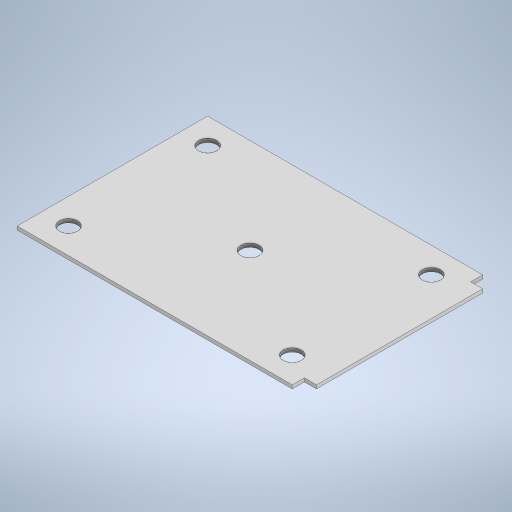
# Autodesk Inventor part: Prateleira
Saved by Autodesk Inventor 2024 (Build 280153000, 153)
## iProperties
Created: 2024-10-14
Part Number: Prateleira
Material: Genérico
Document SubType Name: Modeling
Designer: robof
Density: 1 g/cm^3
Appearance: Padrão
Author: robof
Autodesk Inventor part; units mm, degrees
ref_plane "YZ Plane" through (0, 0, 0) normal (1, 0, 0) x (0, 1, 0)
ref_plane "XZ Plane" through (0, 0, 0) normal (0, 1, 0) x (-1, 0, 0)
ref_plane "XY Plane" through (0, 0, 0) normal (0, 0, 1) x (1, 0, 0)
sketch "Esboço1" plane through (0, 0, 0) normal (0, 1, 0) x (-1, 0, 0)
  line L0 (0, 0) -> (495, 0)
  line L1 (495, 0) -> (495, -315)
  line L2 (495, -315) -> (0, -315)
  line L3 (0, -315) -> (0, 0)
  line L4 (495, 0) -> (475, 0)
  line L5 (475, 0) -> (475, -315)
  line L6 (475, -315) -> (495, -315)
  line L7 (495, -315) -> (495, 0)
  line L8 (0, 0) -> (20, 0)
  line L9 (20, 0) -> (20, -20)
  line L10 (20, -20) -> (0, -20)
  line L11 (0, -20) -> (0, 0)
  line L12 (0, -315) -> (20, -315)
  line L13 (20, -315) -> (20, -295)
  line L14 (20, -295) -> (0, -295)
  line L15 (0, -295) -> (0, -315)
  dimension "d0" = 495
  dimension "d1" = 315
  dimension "d2" = 20
  dimension "d3" = 20
  dimension "d4" = 20
  dimension "d5" = 20
  constraints: 32 end point, 8 parallel, 4 horizontal, 4 perpendicular, 1 point on line
  measures "d0" distance of L1.end L2.end
  measures "d1" distance of L0.end L1.end
  measures "d2" distance of L6.end L5.end
  measures "d3" distance of L9.end L10.end
  measures "d4" distance of L8.end L9.end
  measures "d5" distance of L13.end L12.end
extrude "Extrusão1" add sketch "Esboço1" along normal blind 6 contours L0 L5 L2 L13 L14 L3 L10 L9
sketch "Esboço2" plane through (0, 6, 0) normal (0, 1, 0) x (1, 0, 0)
  line L0 (-475, 315) -> (-475, 0) projected
  line L1 (-475, 315) -> (-432.5736, 272.5736)
  line L2 (-475, 315) -> (-415, 315) construction
  circle A0 centre (-432.5736, 272.5736) radius 15
  line L3 (-475, 157.5) -> (-417.5736, 157.5)
  circle A1 centre (-432.5736, 42.4264) radius 15
  line L4 (-475, 0) -> (-20, 0) projected
  line L5 (-247.5, 0) -> (-247.5, 64.8127)
  circle A2 centre (-62.4264, 272.5736) radius 15
  circle A3 centre (-62.4264, 42.4264) radius 15
  line L6 (-417.5736, 157.5) -> (-161.5581, 157.5)
  line L7 (-247.5, 64.8127) -> (-247.5, 157.5)
  circle A4 centre (-247.5, 157.5) radius 15
  point P0 (0, 0)
  dimension "d8" = 60
  dimension "d9" = 45
  dimension "d10" = 30
  dimension "d11" = 30
  constraints: 12 end point, 5 centre point, 3 horizontal, 3 symmetric about line, 2 coincident, 2 midpoint, 1 equal length, 1 perpendicular, 1 point on line, 1 vertical, 3 other
  measures "d8" distance of L0.start L1.end
  measures "d9" angle of L1 L2
  measures "d10" diameter of A0
  measures "d11" diameter of A4
extrude "Extrusão2" cut sketch "Esboço2" against normal blind 6 contours A0 | A4 L6 | L6 L7 A4 | L6 A4 L7 | A1 | A2 | A3
